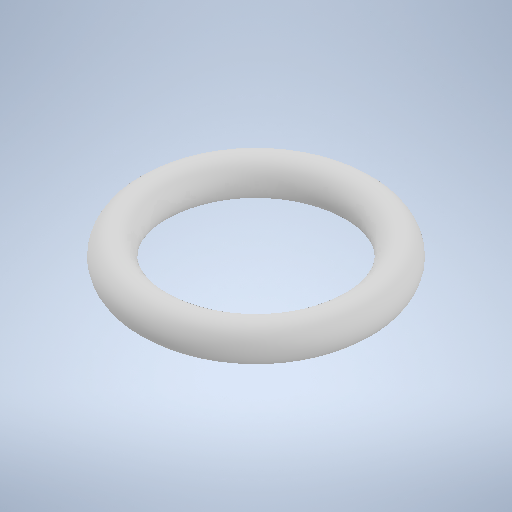
# Autodesk Inventor part: 1_Vòng
Saved by Autodesk Inventor 2025.2 (Build 292293000, 293)
## iProperties
Created: 2024-11-26
Part Number: 1_Vòng
Material: Generic
Document SubType Name: Modeling
Designer: hongquan
Density: 1 g/cm^3
Appearance: Default
Author: hongquan
Autodesk Inventor part; units mm, degrees
ref_plane "YZ Plane" through (0, 0, 0) normal (1, 0, 0) x (0, 1, 0)
ref_plane "XZ Plane" through (0, 0, 0) normal (0, 1, 0) x (-1, 0, 0)
ref_plane "XY Plane" through (0, 0, 0) normal (0, 0, 1) x (1, 0, 0)
sketch "Sketch1" plane through (0, 0, 0) normal (1, 0, 0) x (0, 1, 0)
  line L0 (0, 19.4059) -> (0, -23.313) construction
  circle A0 centre (0, -20) radius 3.5
  line L1 (16.0464, 0) -> (-12.6648, 0)
  point P0 (0, 0)
  dimension "d0" = 7
  dimension "d1" = 20
  constraints: 4 end point, 1 centre point, 1 horizontal, 1 point on line, 1 vertical
  measures "d0" diameter of A0
  measures "d1" distance of A0.centre point (0, 0)
revolve "Revolution1" add sketch "Sketch1" angle 360 about axis through (0, 16.0464, 0) along (0, -1, 0)
body "Solid1"
